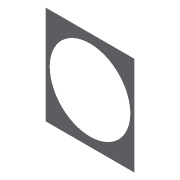
# Autodesk Inventor part: side350x390_hull
Saved by Autodesk Inventor 2014 SP1 (Build 180222100, 222)
## iProperties
Created: 2015-02-11
Part Number: side350x390_hull
Material: Generic
Document SubType Name: Modeling
Designer: Simen
Density: 1 g/cm^3
Appearance: Default
Author: Simen
Autodesk Inventor part; units mm, degrees
ref_plane "YZ Plane" through (0, 0, 0) normal (1, 0, 0) x (0, 1, 0)
ref_plane "XZ Plane" through (0, 0, 0) normal (0, 1, 0) x (-1, 0, 0)
ref_plane "XY Plane" through (0, 0, 0) normal (0, 0, 1) x (1, 0, 0)
sketch "Sketch1" plane through (0, 0, 0) normal (0, 1, 0) x (-1, 0, 0)
  line L0 (-168.1278, 70.4675) -> (181.8722, 70.4675)
  line L1 (181.8722, 70.4675) -> (181.8722, -319.5325)
  line L2 (181.8722, -319.5325) -> (-168.1278, -319.5325)
  line L3 (-168.1278, -319.5325) -> (-168.1278, 70.4675)
  circle A0 centre (6.8722, -124.5325) radius 160
  point P0 (0, 0)
  dimension "d0" = 350
  dimension "d1" = 390
  dimension "d2" = 320
  constraints: 8 end point, 2 parallel, 1 centre point, 1 horizontal, 1 perpendicular
  measures "d0" distance of L1.end L2.end
  measures "d1" distance of L0.end L1.end
  measures "d2" diameter of A0
extrude "Extrusion1" add sketch "Sketch1" along normal blind 0.8
body "Solid1"
